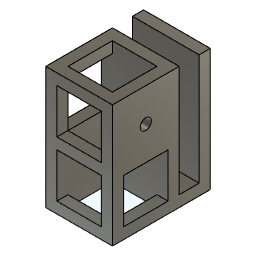
DrzacKamereZaALUFrame v1 (Autodesk Fusion 360 design; units mm, degrees)
Autodesk Fusion 360 part; units mm, degrees
sketch "Sketch1" plane through (0, 0, 0) normal (0, 0, 1) x (1, 0, 0)
  line L0 (25, 75) -> (55, 75)
  line L1 (55, 75) -> (55, 45)
  line L2 (55, 45) -> (25, 45)
  line L3 (25, 45) -> (25, 75)
  dimension "d1" = 30
  dimension "d2" = 30
  constraint horizontal L0
  constraint vertical L1
  constraint horizontal L2
  constraint vertical L3
  measures "d1" distance of L0.start L0.end
  measures "d2" distance of L0.start L2.end
extrude "Extrude1" add sketch "Sketch1" along normal blind 55
sketch "Sketch2" plane through (0, 0, 0) normal (0, 0, 1) x (1, 0, 0)
  line L0 (25, 75) -> (25, 70)
  line L1 (25, 70) -> (50, 70)
  line L2 (50, 70) -> (50, 50)
  line L3 (50, 50) -> (30, 50)
  line L4 (30, 50) -> (30, 70)
  dimension "d5" = 5
  dimension "d6" = 25
  dimension "d7" = 20
  dimension "d8" = 20
  constraint vertical L0
  constraint perpendicular L0 L1
  constraint perpendicular L1 L2
  constraint perpendicular L2 L3
  constraint coincident L1 L4.end
  constraint perpendicular L1 L4
  measures "d5" distance of L0.start L0.end
  measures "d6" distance of L0.end L1.end
  measures "d7" distance of L1.end L2.end
  measures "d8" distance of L2.end L3.end
extrude "Extrude2" cut sketch "Sketch2" along normal blind 55
sketch "Sketch3" plane through (25, 0, 0) normal (-1, 0, 0) x (0, -1, 0)
  line L0 (-75, 0) -> (-45, 0)
  line L1 (-45, 0) -> (-45, 55)
  line L2 (-45, 55) -> (-75, 55)
  line L3 (-75, 55) -> (-75, 0)
  line L4 (-70, 50) -> (-50, 50)
  line L5 (-50, 50) -> (-50, 30)
  line L6 (-50, 30) -> (-70, 30)
  line L7 (-70, 30) -> (-70, 50)
  line L8 (-70, 25) -> (-50, 25)
  line L9 (-50, 25) -> (-50, 5)
  line L10 (-50, 5) -> (-70, 5)
  line L11 (-70, 5) -> (-70, 25)
  constraint horizontal L4
  constraint perpendicular L4 L5
  constraint perpendicular L5 L6
  constraint perpendicular L4 L7
  constraint perpendicular L7 L8
  constraint perpendicular L6 L9
  constraint perpendicular L9 L10
  constraint perpendicular L8 L11
extrude "Extrude3" cut sketch "Sketch3" against normal blind 6 contours L4 L5 L6 L7 | L8 L9 L10 L11
sketch "Sketch4" plane through (0, 45, 0) normal (0, -1, 0) x (1, 0, 0)
  line L0 (25, 0) -> (55, 0)
  line L1 (55, 0) -> (55, 55)
  line L2 (55, 55) -> (25, 55)
  line L3 (25, 55) -> (25, 0)
  line L4 (30, 50) -> (50, 50)
  line L5 (50, 50) -> (50, 30)
  line L6 (50, 30) -> (30, 30)
  line L7 (30, 50) -> (30, 30)
  line L8 (30, 25) -> (50, 25)
  line L9 (50, 25) -> (50, 5)
  line L10 (50, 5) -> (30, 5)
  line L11 (30, 5) -> (30, 25)
  constraint perpendicular L3 L4
  constraint perpendicular L4 L5
  constraint perpendicular L3 L6
  constraint perpendicular L4 L7
  constraint perpendicular L3 L8
  constraint perpendicular L4 L9
  constraint perpendicular L9 L10
  constraint perpendicular L4 L11
extrude "Extrude4" cut sketch "Sketch4" against normal blind 5 contours L4 L5 L6 L7 | L8 L9 L10 L11
sketch "Sketch5" plane through (55, 0, 0) normal (1, 0, 0) x (0, 1, 0)
  line L0 (45, 0) -> (75, 0)
  line L1 (75, 0) -> (75, 55)
  line L2 (75, 55) -> (45, 55)
  line L3 (45, 55) -> (45, 0)
  line L4 (50, 50) -> (70, 50)
  line L5 (70, 50) -> (70, 30)
  line L6 (70, 30) -> (50, 30)
  line L7 (50, 30) -> (50, 50)
  line L8 (50, 25) -> (70, 25)
  line L9 (70, 25) -> (70, 5)
  line L10 (70, 5) -> (50, 5)
  line L11 (50, 5) -> (50, 25)
  constraint perpendicular L3 L4
  constraint perpendicular L2 L5
  constraint perpendicular L3 L6
  constraint perpendicular L4 L7
  constraint perpendicular L7 L8
  constraint perpendicular L6 L9
  constraint perpendicular L7 L10
  constraint perpendicular L8 L11
extrude "Extrude5" cut sketch "Sketch5" against normal blind 5 contours L4 L5 L6 L7 | L8 L9 L10 L11
sketch "Sketch6" plane through (0, 0, 0) normal (0, 0, -1) x (1, 0, 0)
  line L0 (30, -70) -> (30, -50)
  line L1 (30, -50) -> (50, -50)
  line L2 (50, -50) -> (50, -70)
  line L3 (50, -70) -> (30, -70)
  line L4 (55, -45) -> (25, -45)
  line L5 (25, -45) -> (25, -75)
  line L6 (25, -75) -> (55, -75)
  line L7 (55, -75) -> (55, -45)
sketch "Sketch7" plane through (55, 0, 0) normal (1, 0, 0) x (0, 1, 0)
  line L0 (70, 50) -> (70, 30)
  line L1 (70, 30) -> (50, 30)
  line L2 (50, 30) -> (50, 50)
  line L3 (50, 50) -> (70, 50)
  line L4 (70, 25) -> (70, 5)
  line L5 (70, 5) -> (50, 5)
  line L6 (50, 5) -> (50, 25)
  line L7 (50, 25) -> (70, 25)
  line L8 (45, 0) -> (75, 0)
  line L9 (75, 0) -> (75, 55)
  line L10 (75, 55) -> (45, 55)
  line L11 (45, 55) -> (45, 0)
  line L12 (75, 0) -> (84, 0)
  line L13 (84, 0) -> (89, 0)
  line L14 (84, 0) -> (84, 55)
  line L15 (84, 55) -> (89, 55)
  line L16 (89, 55) -> (89, 0)
  line L17 (75, 0) -> (75, 5)
  line L18 (75, 5) -> (84, 5)
  dimension "d17" = 9
  dimension "d18" = 5
  dimension "d19" = 5
  constraint coincident L8.end L9.start
  constraint perpendicular L9 L12
  constraint parallel L12 L13
  constraint perpendicular L13 L14
  constraint perpendicular L14 L15
  constraint coincident L9 L17.end
  constraint perpendicular L12 L17
  constraint coincident L14 L18.end
  constraint perpendicular L14 L18
  measures "d17" distance of L8.end L12.end
  measures "d18" distance of L12.end L13.end
  measures "d19" distance of L14.end L15.end
extrude "Extrude6" add sketch "Sketch7" against normal blind 30 contours L9 L12 L14 L17 L18 | L13 L14 L15 L16
sketch "Sketch8" plane through (0, 0, 0) normal (1, 0, 0) x (0, 1, 0)
sketch "Sketch9" plane through (25, 0, 0) normal (-1, 0, 0) x (0, -1, 0)
  line L0 (-50, 50) -> (-50, 30)
  line L1 (-50, 30) -> (-70, 30)
  line L2 (-70, 30) -> (-70, 50)
  line L3 (-70, 50) -> (-50, 50)
  line L4 (-50, 25) -> (-50, 5)
  line L5 (-50, 5) -> (-70, 5)
  line L6 (-70, 5) -> (-70, 25)
  line L7 (-70, 25) -> (-50, 25)
  line L8 (-89, 0) -> (-45, 0)
  line L9 (-45, 0) -> (-45, 55)
  line L10 (-45, 55) -> (-75, 55)
  line L11 (-75, 55) -> (-75, 5)
  line L12 (-75, 5) -> (-84, 5)
  line L13 (-84, 5) -> (-84, 55)
  line L14 (-84, 55) -> (-89, 55)
  line L15 (-89, 55) -> (-89, 0)
  line L16 (-50, 5) -> (-70, 5)
  line L17 (-70, 5) -> (-70, 25)
  line L18 (-70, 25) -> (-50, 25)
  line L19 (-50, 25) -> (-50, 5)
  constraint horizontal L16
  constraint vertical L17
  constraint horizontal L18
  constraint vertical L19
  constraint coincident L6.end L7.start
  constraint coincident L4.end L5.start
extrude "Extrude7" add sketch "Sketch9" against normal blind 5 contours L4 L5 L6 L7 L16 L17 L18 L19
sketch "Sketch10" plane through (25, 0, 0) normal (-1, 0, 0) x (0, -1, 0)
  line L0 (-50, 50) -> (-50, 30)
  line L1 (-50, 30) -> (-70, 30)
  line L2 (-70, 30) -> (-70, 50)
  line L3 (-70, 50) -> (-50, 50)
  line L4 (-89, 0) -> (-45, 0)
  line L5 (-45, 0) -> (-45, 55)
  line L6 (-45, 55) -> (-75, 55)
  line L7 (-75, 55) -> (-75, 5)
  line L8 (-75, 5) -> (-84, 5)
  line L9 (-84, 5) -> (-84, 55)
  line L10 (-84, 55) -> (-89, 55)
  line L11 (-89, 55) -> (-89, 0)
  line L12 (-60, 0) -> (-60, 15)
  circle A0 centre (-60, 15) radius 2.5
  dimension "d24" = 5
  constraint coincident L4 L12.start
  constraint perpendicular L4 L12
  constraint coincident L12.end A0.centre
  measures "d24" diameter of A0
extrude "Extrude8" cut sketch "Sketch10" against normal blind 5 contours A0
sketch "Sketch11" plane through (55, 0, 0) normal (1, 0, 0) x (0, 1, 0)
  line L0 (70, 50) -> (70, 30)
  line L1 (70, 30) -> (50, 30)
  line L2 (50, 30) -> (50, 50)
  line L3 (50, 50) -> (70, 50)
  line L4 (70, 25) -> (70, 5)
  line L5 (70, 5) -> (50, 5)
  line L6 (50, 5) -> (50, 25)
  line L7 (50, 25) -> (70, 25)
  line L8 (45, 0) -> (89, 0)
  line L9 (89, 0) -> (89, 55)
  line L10 (89, 55) -> (84, 55)
  line L11 (84, 55) -> (84, 5)
  line L12 (84, 5) -> (75, 5)
  line L13 (75, 5) -> (75, 55)
  line L14 (75, 55) -> (45, 55)
  line L15 (45, 55) -> (45, 0)
  line L16 (70, 30) -> (50, 30)
  line L17 (50, 30) -> (50, 50)
  line L18 (50, 50) -> (70, 50)
  line L19 (70, 50) -> (70, 30)
  constraint horizontal L16
  constraint vertical L17
  constraint horizontal L18
  constraint vertical L19
  constraint coincident L2.end L3.start
  constraint coincident L0.end L1.start
extrude "Extrude9" add sketch "Sketch11" against normal blind 5 contours L0 L1 L2 L3 L16 L17 L18 L19
sketch "Sketch12" plane through (55, 0, 0) normal (1, 0, 0) x (0, 1, 0)
  line L0 (70, 25) -> (70, 5)
  line L1 (70, 5) -> (50, 5)
  line L2 (50, 5) -> (50, 25)
  line L3 (50, 25) -> (70, 25)
  line L4 (45, 0) -> (89, 0)
  line L5 (89, 0) -> (89, 55)
  line L6 (89, 55) -> (84, 55)
  line L7 (84, 55) -> (84, 5)
  line L8 (84, 5) -> (75, 5)
  line L9 (75, 5) -> (75, 55)
  line L10 (75, 55) -> (45, 55)
  line L11 (45, 55) -> (45, 0)
  line L12 (60, 55) -> (60, 40)
  circle A0 centre (60, 40) radius 2.5
  dimension "d29" = 5
  constraint midpoint L10 L12.start
  constraint perpendicular L10 L12
  constraint coincident L12.end A0.centre
  measures "d29" diameter of A0
extrude "Extrude10" cut sketch "Sketch12" against normal blind 5 contours A0
